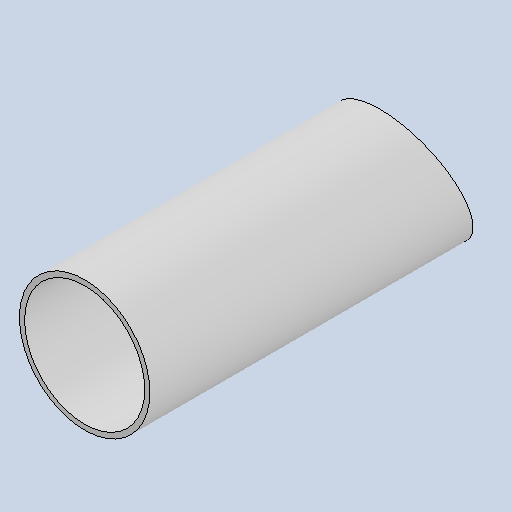
# Autodesk Inventor part: MSC 606 rocket tube 6
Saved by Autodesk Inventor 2025 (Build 290162010, 162A)
## iProperties
Created: 2024-05-24
Part Number: MSC 606 rocket tube 6
Material: Generic
Document SubType Name: Modeling
Designer: admin
Density: 1 g/cm^3
Appearance: Default
Stock Number: МОО 606 ракета труба 6
Author: admin
Autodesk Inventor part; units mm, degrees
ref_plane "YZ Plane" through (0, 0, 0) normal (1, 0, 0) x (0, 1, 0)
ref_plane "XZ Plane" through (0, 0, 0) normal (0, 1, 0) x (-1, 0, 0)
ref_plane "XY Plane" through (0, 0, 0) normal (0, 0, 1) x (1, 0, 0)
sketch "Sketch1" plane through (0, 0, 0) normal (0, 0, 1) x (1, 0, 0)
  circle A0 centre (0, 0) radius 38.05
  circle A1 centre (0, 0) radius 35.05
  dimension "d0" = 76.1
  dimension "d1" = 3
  constraints: 2 centre point, 1 coincident
  measures "d0" diameter of A0
  measures "d1" radial gap between concentric circles of A0 A1
extrude "Extrusion1" add sketch "Sketch1" along normal blind 200
sketch "Sketch2" plane through (0, 0, 0) normal (1, 0, 0) x (0, 1, 0)
  line L0 (38.05, 200) -> (-38.05, 200) projected
  line L1 (38.05, 0) -> (-38.05, 0) projected
  line L2 (-38.05, 0) -> (38.05, 27.6981)
  line L3 (38.05, 27.6981) -> (38.05, 0)
  line L4 (38.05, 0) -> (38.05, 200) projected
  point P0 (0, 0)
  dimension "d4" = 20
  constraints: 4 end point, 1 collinear
  measures "d4" angle of L2 L1
extrude "Extrusion2" cut sketch "Sketch2" along normal mid plane 300
body "Solid1"
